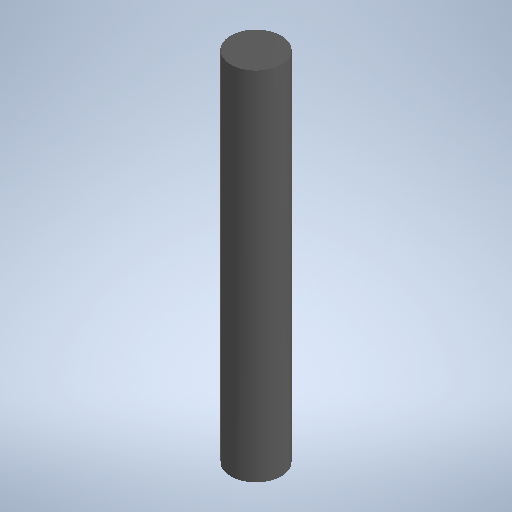
# Autodesk Inventor part: Long_removable_nose_peg
Saved by Autodesk Inventor 2025.1 (Build 291241020, 241B)
## iProperties
Part Number: Long_removable_nose_peg
Material: Generic
Document SubType Name: Modeling
Designer: smyth
Appearance: Default
Author: smyth
Autodesk Inventor part; units mm, degrees
ref_plane "YZ Plane" through (0, 0, 0) normal (1, 0, 0) x (0, 1, 0)
ref_plane "XZ Plane" through (0, 0, 0) normal (0, 1, 0) x (-1, 0, 0)
ref_plane "XY Plane" through (0, 0, 0) normal (0, 0, 1) x (1, 0, 0)
sketch "Sketch1" plane through (0, 0, 0) normal (0, 1, 0) x (-1, 0, 0)
  circle A0 centre (0, 0) radius 1.2375
  dimension "d0" = 2.475
  constraints: 1 centre point, 1 coincident
  measures "d0" diameter of A0
extrude "Extrusion1" add sketch "Sketch1" along normal blind 17.5
body "Solid1"
